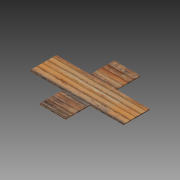
# Autodesk Inventor part: Electronics Board
Saved by Autodesk Inventor 2015 SP1 (Build 190203100, 203)
## iProperties
Created: 2015-01-27
Part Number: Electronics Board
Material: Generic
Document SubType Name: Modeling
Designer: pltwe4
Density: 1 g/cm^3
Appearance: Wood - Batten New
Author: pltwe4
Autodesk Inventor part; units mm, degrees
ref_plane "YZ Plane" through (0, 0, 0) normal (1, 0, 0) x (0, 1, 0)
ref_plane "XZ Plane" through (0, 0, 0) normal (0, 1, 0) x (-1, 0, 0)
ref_plane "XY Plane" through (0, 0, 0) normal (0, 0, 1) x (1, 0, 0)
sketch "Sketch1" plane through (0, 0, 0) normal (0, 1, 0) x (-1, 0, 0)
  line L0 (88.9, 254) -> (-88.9, 254)
  line L1 (-88.9, -254) -> (88.9, -254)
  line L2 (0, -266.7) -> (0, 266.7) projected
  line L3 (-444.5, 0) -> (444.5, 0) projected
  line L4 (88.9, -88.9) -> (317.5, -88.9)
  line L5 (317.5, -88.9) -> (317.5, 88.9)
  line L6 (317.5, 88.9) -> (88.9, 88.9)
  line L7 (-88.9, 88.9) -> (-317.5, 88.9)
  line L8 (-317.5, 88.9) -> (-317.5, -88.9)
  line L9 (-317.5, -88.9) -> (-88.9, -88.9)
  line L10 (88.9, -254) -> (88.9, -88.9)
  line L11 (88.9, 88.9) -> (88.9, 254)
  line L12 (-88.9, 254) -> (-88.9, 88.9)
  line L13 (-88.9, -88.9) -> (-88.9, -254)
  line L14 (88.9, -88.9) -> (88.9, 88.9)
  line L15 (-88.9, -88.9) -> (-88.9, 88.9)
  line L16 (88.9, -88.9) -> (-88.9, -88.9)
  line L17 (-88.9, 88.9) -> (88.9, 88.9)
  point P0 (0, 0)
  dimension "d1" = 177.8
  dimension "d5" = 177.8
  dimension "d6" = 635
  dimension "d7" = 508
  constraints: 32 end point, 8 perpendicular, 5 parallel, 2 horizontal, 1 collinear, 1 point on line, 1 vertical, 8 other
  measures "d1" distance of L1.start L1.end
  measures "d5" distance of L7.end L8.end
  measures "d6" distance between parallel lines of L8 L5
  measures "d7" distance between parallel lines of L0 L1
extrude "Extrusion1" add sketch "Sketch1" along normal blind 6.35
equation "\"d1\" = Height"
equation "\"d5\" = Width"
equation "\"d6\" = HLength"
equation "\"d7\" = WLength"
equation "\"HLength\" = 635"
equation "\"Height\" = 177.8"
equation "\"Width\" = 177.8"
equation "\"WLength\" = 508"
body "Solid1"
